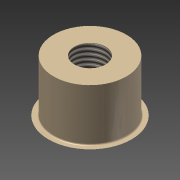
# Autodesk Inventor part: Zaślepka_do_widelca
Saved by Autodesk Inventor 2015 (Build 190159000, 159)
## iProperties
Created: 2016-01-12
Part Number: Zaślepka_do_widelca
Material: Polietylen o dużej gęstości
Document SubType Name: Modeling
Designer: graaapsik
Density: 0.952 g/cm^3
Appearance: Gładki - w kolorze złamanej bieli
Author: graaapsik
Autodesk Inventor part; units mm, degrees
ref_plane "YZ Plane" through (0, 0, 0) normal (1, 0, 0) x (0, 1, 0)
ref_plane "XZ Plane" through (0, 0, 0) normal (0, 1, 0) x (-1, 0, 0)
ref_plane "XY Plane" through (0, 0, 0) normal (0, 0, 1) x (1, 0, 0)
sketch "Szkic1" plane through (0, 0, 0) normal (0, 0, 1) x (1, 0, 0)
  circle A0 centre (0, 0) radius 14
  dimension "d0" = 28
  constraints: 1 centre point, 1 coincident
  measures "d0" diameter of A0
extrude "Wyciągnięcie proste1" add sketch "Szkic1" along normal blind 20
shell "Skorupa1" thickness 8 removed faces 2 at (0.5625, 1.5565, 20) at (0.5625, 1.5565, 0)
sketch "Szkic2" plane through (0, 0, 0) normal (0, 1, 0) x (-1, 0, 0)
  line L0 (-14, 0) -> (14, 0) construction
  line L1 (0, 0) -> (16, 0)
  line L2 (0, 0) -> (0, -3)
  arc A0 (0, -3) -> (16, 0) centre (0, 41.1667) ccw
  dimension "d4" = 16
  dimension "d5" = 3
  constraints: 4 end point, 2 point on circle, 1 centre point, 1 collinear, 1 line through centre, 1 perpendicular
  measures "d4" distance from line of L1.end L2
  measures "d5" distance of L1.start L2.end
revolve "Obrót1" add sketch "Szkic2" angle 360 about axis through (0, 0, 0) along (0, 0, -1)
fillet "Zaokrąglenie1" radius 0.5 1 edges at (-14, 0, 0)
thread "Gwint1" size "M12x1.75" class "6H" standard "ANSI Metric M Profile" full length
